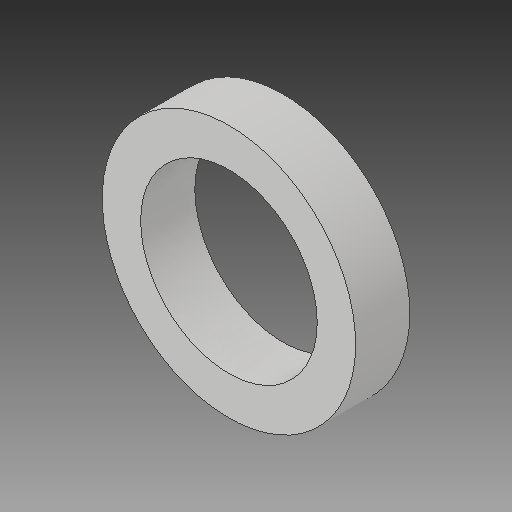
# Autodesk Inventor part: distance_short
Saved by Autodesk Inventor 2019.3 (Build 233278000, 278)
## iProperties
Created: 2020-08-26
Part Number: distance_short
Material: Generisch
Document SubType Name: Modeling
Designer: Nicolas Frick
Density: 1 g/cm^3
Appearance: Vorgabe
Mass: 0.138363 g
Surface Area: 2.66592 cm^2
Volume: 0.138363 cm^3
Author: Nicolas Frick
Autodesk Inventor part; units mm, degrees
ref_plane "YZ Plane" through (0, 0, 0) normal (1, 0, 0) x (0, 1, 0)
ref_plane "XZ Plane" through (0, 0, 0) normal (0, 1, 0) x (-1, 0, 0)
ref_plane "XY Plane" through (0, 0, 0) normal (0, 0, 1) x (1, 0, 0)
sketch "Skizze1" plane through (0, 0, 0) normal (0, 0, 1) x (1, 0, 0)
  circle A0 centre (0, 0) radius 3.9902 construction
  circle A1 centre (0, 0) radius 5.35 construction
  circle A2 centre (0, 0) radius 4.075
  circle A3 centre (0, 0) radius 5.85
  dimension "d2" = 8.15
  dimension "d3" = 11.7
  constraints: 2 centre point, 2 coincident
  measures "d2" diameter of A2
  measures "d3" diameter of A3
extrude "Extrusion2" add sketch "Skizze1" along normal blind 2.5
